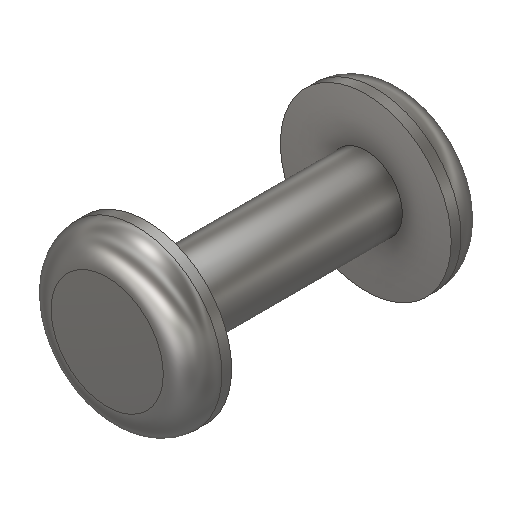
# Autodesk Inventor part: CNCT_STEEL_Bucket_tooth_mounting_pin
Saved by Autodesk Inventor 2025 (Build 290162010, 162A)
## iProperties
Created: 2018-09-17
Part Number: CNCT_STEEL_Bucket_tooth_mounting_pin
Material: Stainless Steel
Document SubType Name: Modeling
Designer: Andrzej
Density: 8 g/cm^3
Appearance: Semi-Polished
Mass: 0.174217 g
Surface Area: 0.677654 cm^2
Volume: 0.0217771 cm^3
Author: Andrzej
Autodesk Inventor part; units mm, degrees
ref_plane "YZ Plane" through (0, 0, 0) normal (1, 0, 0) x (0, 1, 0)
ref_plane "XZ Plane" through (0, 0, 0) normal (0, 1, 0) x (-1, 0, 0)
ref_plane "XY Plane" through (0, 0, 0) normal (0, 0, 1) x (1, 0, 0)
sketch "Sketch1" plane through (0, 0, 0) normal (0, 0, 1) x (1, 0, 0)
  circle A0 centre (0, 0) radius 0.75
  circle A1 centre (0, 0) radius 1.75
  dimension "d0" = 1.5
  dimension "d3" = 1
  constraints: 2 centre point, 1 coincident
  measures "d0" diameter of A0
  measures "d3" radial gap between concentric circles of A0 A1
extrude "Extrusion1" add sketch "Sketch1" along normal blind 4.5 contours A0
extrude "Extrusion2" add sketch "Sketch1" against normal blind 0.8 contours A0 | A1
sketch "Sketch2" plane through (0, 0, 4.5) normal (0, 0, 1) x (1, 0, 0)
  circle A0 centre (0, 0) radius 1.75 projected
  circle A1 centre (0, 0) radius 0.75 projected
extrude "Extrusion3" add sketch "Sketch2" along normal blind 0.8 contours A0 | A1
fillet "Fillet1" radius 0.6 2 edges at (-1.75, 0, 5.3) (-1.75, 0, -0.8)
body "Solid1"
